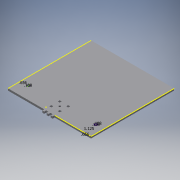
# Autodesk Inventor part: Part7
Saved by Autodesk Inventor 2018 (Build 220112000, 112)
## iProperties
Created: 2018-04-30
Part Number: Part7
Material: Generic
Document SubType Name: Modeling
Designer: Administrator
Density: 1 g/cm^3
Appearance: Default
Mass: 196.452 g
Surface Area: 869.407 cm^2
Volume: 196.452 cm^3
Author: Administrator
Autodesk Inventor part; units mm, degrees
ref_plane "YZ Plane" through (0, 0, 0) normal (1, 0, 0) x (0, 1, 0)
ref_plane "XZ Plane" through (0, 0, 0) normal (0, 1, 0) x (-1, 0, 0)
ref_plane "XY Plane" through (0, 0, 0) normal (0, 0, 1) x (1, 0, 0)
sketch "Sketch1" plane through (0, 0, 0) normal (0, 1, 0) x (-1, 0, 0)
  line L0 (86.6175, 6.5548) -> (-116.5825, 6.5548)
  line L1 (-116.5825, 6.5548) -> (-116.5825, -196.6452)
  line L2 (-116.5825, -196.6452) -> (86.6175, -196.6452)
  line L3 (86.6175, -196.6452) -> (86.6175, 6.5548)
  point P0 (0, 0)
  dimension "d0" = 203.2
  dimension "d1" = 203.2
  constraints: 8 end point, 2 parallel, 1 horizontal, 1 perpendicular
  measures "d0" distance between parallel lines of L1 L3
  measures "d1" distance between parallel lines of L2 L0
extrude "Extrusion1" add sketch "Sketch1" along normal blind 4.7625
sketch "Sketch4" plane through (-86.6175, 0, 6.5548) normal (0, 0, 1) x (1, 0, 0)
  line L0 (0, 0) -> (203.2, 0) projected
  line L1 (0, 4.7625) -> (203.2, 4.7625) projected
  line L2 (88.9, 0) -> (93.6625, 0)
  line L3 (93.6625, 0) -> (93.6625, 4.7625)
  line L4 (93.6625, 4.7625) -> (88.9, 4.7625)
  line L5 (88.9, 4.7625) -> (88.9, 0)
  line L6 (99.2188, 0) -> (103.9813, 0)
  line L7 (103.9813, 0) -> (103.9813, 4.7625)
  line L8 (103.9813, 4.7625) -> (99.2188, 4.7625)
  line L9 (99.2188, 4.7625) -> (99.2188, 0)
  line L10 (109.5375, 4.7625) -> (114.3, 4.7625)
  line L11 (114.3, 4.7625) -> (114.3, 0)
  line L12 (114.3, 0) -> (109.5375, 0)
  line L13 (109.5375, 0) -> (109.5375, 4.7625)
  line L14 (0, 0) -> (0, 4.7625) projected
  point P0 (86.6175, 0)
  dimension "d12" = 4.7625
  dimension "d13" = 4.7625
  dimension "d14" = 5.5563
  dimension "d15" = 4.7625
  dimension "d16" = 5.5563
  dimension "d17" = 88.9
  constraints: 24 end point, 6 parallel, 6 point on line, 3 horizontal, 3 perpendicular
  measures "d12" distance between parallel lines of L3 L5
  measures "d13" distance between parallel lines of L7 L9
  measures "d14" distance between parallel lines of L3 L9
  measures "d15" distance between parallel lines of L11 L13
  measures "d16" distance between parallel lines of L7 L13
  measures "d17" distance between parallel lines of L5 L14
extrude "Extrusion3" add sketch "Sketch4" along normal blind 4.7625 contours L5 L1 L3 L0 | L9 L1 L7 L0 | L13 L1 L11 L0
sketch "Sketch5" plane through (0, 4.7625, 0) normal (0, 1, 0) x (1, 0, 0)
  line L0 (22.92, 10.9077) -> (27.6825, 10.9077)
  line L1 (27.6825, 10.9077) -> (27.6825, 6.1452)
  line L2 (27.6825, 6.1452) -> (22.92, 6.1452)
  line L3 (22.92, 6.1452) -> (22.92, 10.9077)
  line L4 (17.3637, -6.5548) -> (22.92, -6.5548) projected
  line L5 (7.045, 6.1452) -> (2.2825, 6.1452)
  line L6 (2.2825, 6.1452) -> (2.2825, 10.9077)
  line L7 (2.2825, 10.9077) -> (7.045, 10.9077)
  line L8 (7.045, 10.9077) -> (7.045, 6.1452)
  line L9 (116.5825, -6.5548) -> (116.5825, 196.6452) projected
  line L10 (22.92, 26.7827) -> (27.6825, 26.7827)
  line L11 (27.6825, 26.7827) -> (27.6825, 31.5452)
  line L12 (27.6825, 31.5452) -> (22.92, 31.5452)
  line L13 (22.92, 31.5452) -> (22.92, 26.7827)
  line L14 (7.045, 26.7827) -> (2.2825, 26.7827)
  line L15 (2.2825, 26.7827) -> (2.2825, 31.5452)
  line L16 (2.2825, 31.5452) -> (7.045, 31.5452)
  line L17 (7.045, 31.5452) -> (7.045, 26.7827)
  point P0 (0, 0)
  dimension "d20" = 4.7625
  dimension "d21" = 4.7625
  dimension "d22" = 12.7
  dimension "d23" = 4.7625
  dimension "d24" = 15.875
  dimension "d25" = 88.9
  dimension "d26" = 4.7625
  dimension "d27" = 15.875
  constraints: 32 end point, 8 parallel, 4 horizontal, 4 perpendicular
  measures "d20" distance between parallel lines of L0 L2
  measures "d21" distance between parallel lines of L3 L1
  measures "d22" distance between parallel lines of L4 L2
  measures "d23" distance between parallel lines of L8 L6
  measures "d24" distance between parallel lines of L3 L8
  measures "d25" distance between parallel lines of L9 L1
  measures "d26" distance between parallel lines of L12 L10
  measures "d27" distance between parallel lines of L0 L10
extrude "Extrusion4" cut sketch "Sketch5" against normal blind 4.7625
sketch "Sketch6" plane through (0, 4.7625, 0) normal (0, 1, 0) x (1, 0, 0)
  line L0 (22.92, 6.1452) -> (22.92, 10.9077) projected
  line L1 (27.6825, 26.7827) -> (22.92, 26.7827) projected
  point P0 (0, 0)
  point P1 (14.9825, 18.8452)
  dimension "d30" = 7.9375
  dimension "d31" = 7.9375
  measures "d30" distance from line of L0 point (14.982, 18.845)
  measures "d31" distance from line of L1 point (14.982, 18.845)
hole "Hole1" at (14.9825, 4.7625, -18.8452) direction (0, -1, 0) diameter 4.7625 depth 25.4 tip angle 118
sketch "Sketch7" plane through (0, 4.7625, 0) normal (0, 1, 0) x (1, 0, 0)
  line L0 (95.1512, 26.7827) -> (99.9137, 26.7827)
  line L1 (99.9137, 26.7827) -> (99.9137, 22.0202)
  line L2 (99.9137, 22.0202) -> (95.1512, 22.0202)
  line L3 (95.1512, 22.0202) -> (95.1512, 26.7827)
  line L4 (116.5825, -6.5548) -> (116.5825, 196.6452) projected
  line L5 (27.6825, -6.5548) -> (116.5825, -6.5548) projected
  line L6 (-65.1863, 22.0202) -> (-69.9488, 22.0202)
  line L7 (-69.9488, 22.0202) -> (-69.9488, 26.7827)
  line L8 (-69.9488, 26.7827) -> (-65.1863, 26.7827)
  line L9 (-65.1863, 26.7827) -> (-65.1863, 22.0202)
  line L10 (-86.6175, 196.6452) -> (-86.6175, -6.5548) projected
  line L11 (8.2581, 103.7764) -> (13.0206, 103.7764)
  line L12 (13.0206, 103.7764) -> (13.0206, 99.0139)
  line L13 (13.0206, 99.0139) -> (8.2581, 99.0139)
  line L14 (8.2581, 99.0139) -> (8.2581, 103.7764)
  point P0 (0, 0)
  dimension "d39" = 4.7625
  dimension "d40" = 16.6687
  dimension "d41" = 28.575
  dimension "d42" = 4.7625
  dimension "d43" = 4.7625
  dimension "d44" = 16.6687
  dimension "d45" = 4.7625
  dimension "d46" = 105.5687
  dimension "d47" = 4.7625
  constraints: 24 end point, 6 parallel, 3 horizontal, 3 perpendicular
  measures "d39" distance between parallel lines of L3 L1
  measures "d40" distance between parallel lines of L4 L1
  measures "d41" distance between parallel lines of L5 L2
  measures "d42" distance between parallel lines of L0 L2
  measures "d43" distance between parallel lines of L9 L7
  measures "d44" distance between parallel lines of L10 L7
  measures "d45" distance between parallel lines of L13 L11
  measures "d46" distance between parallel lines of L5 L13
  measures "d47" distance between parallel lines of L14 L12
body "Solid1"
